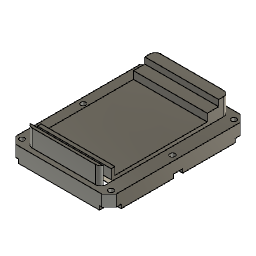
1006315G-Modified (Autodesk Fusion 360 design; units mm, degrees)
Autodesk Fusion 360 part; units mm, degrees
sketch "Sketch1" plane through (0, 0, 0) normal (0, 0, 1) x (1, 0, 0)
  line L0 (6.096, 0) -> (78.105, 0)
  line L1 (84.201, 6.096) -> (84.201, 109.9566)
  line L2 (78.105, 116.0526) -> (6.096, 116.0526)
  line L3 (0, 109.9566) -> (0, 6.096)
  line L4 (6.096, 116.0526) -> (0, 109.9566)
  line L5 (84.201, 109.9566) -> (78.105, 116.0526)
  line L6 (6.096, 0) -> (0, 6.096)
  line L7 (78.105, 0) -> (84.201, 6.096)
  line L8 (93.6149, 58.0263) -> (74.7871, 58.0263) construction
  line L9 (74.7871, 58.0263) -> (-7.9105, 58.0263) construction
  line L10 (91.1489, 109.5883) -> (-7.9105, 109.5883) construction
  line L11 (91.1489, 6.4643) -> (-4.9152, 6.4643) construction
  line L12 (42.1005, 123.6479) -> (42.1005, 108.4573) construction
  line L13 (42.1005, 108.4573) -> (42.1005, -5.2893) construction
  line L14 (79.4385, 120.5753) -> (79.4385, -5.6753) construction
  line L15 (4.7625, 120.9613) -> (4.7625, -5.2893) construction
  circle A0 centre (4.7625, 57.836) radius 2.159
  circle A1 centre (79.4385, 109.5883) radius 2.159
  circle A2 centre (4.7625, 109.5883) radius 2.159
  circle A3 centre (4.7625, 6.4643) radius 2.159
  circle A4 centre (79.4385, 6.4643) radius 2.159
  line L16 (15.4178, 111.887) -> (68.7578, 111.887)
  line L17 (73.0758, 107.569) -> (73.0758, 8.509)
  line L18 (68.7578, 4.191) -> (15.4178, 4.191)
  line L19 (11.0998, 8.509) -> (11.0998, 107.569)
  arc A5 (15.4178, 111.887) -> (11.0998, 107.569) centre (15.4178, 107.569) ccw
  arc A6 (73.0758, 107.569) -> (68.7578, 111.887) centre (68.7578, 107.569) ccw
  arc A7 (11.0998, 8.509) -> (15.4178, 4.191) centre (15.4178, 8.509) ccw
  arc A8 (68.7578, 4.191) -> (73.0758, 8.509) centre (68.7578, 8.509) ccw
  line L20 (0, 61.8363) -> (6.35, 61.8363)
  line L21 (8.89, 59.2963) -> (8.89, 56.7563)
  line L22 (6.35, 54.2163) -> (0, 54.2163)
  line L23 (0, 54.2163) -> (0, 61.8363)
  arc A9 (8.89, 59.2963) -> (6.35, 61.8363) centre (6.35, 59.2963) ccw
  arc A10 (6.35, 54.2163) -> (8.89, 56.7563) centre (6.35, 56.7563) ccw
  line L24 (84.201, 54.2163) -> (77.851, 54.2163)
  line L25 (75.311, 56.7563) -> (75.311, 59.2963)
  line L26 (77.851, 61.8363) -> (84.201, 61.8363)
  line L27 (84.201, 61.8363) -> (84.201, 54.2163)
  circle A11 centre (79.4385, 58.0263) radius 2.159
  arc A12 (77.851, 61.8363) -> (75.311, 59.2963) centre (77.851, 59.2963) ccw
  arc A13 (75.311, 56.7563) -> (77.851, 54.2163) centre (77.851, 56.7563) ccw
  line L28 (76.073, 0) -> (84.201, 0)
  line L29 (84.201, 0) -> (84.201, 10.16)
  line L30 (84.201, 10.16) -> (78.613, 10.16)
  line L31 (76.073, 7.62) -> (76.073, 0)
  arc A14 (78.613, 10.16) -> (76.073, 7.62) centre (78.613, 7.62) ccw
  line L32 (8.128, 0) -> (0, 0)
  line L33 (0, 0) -> (0, 10.16)
  line L34 (0, 10.16) -> (5.588, 10.16)
  line L35 (8.128, 7.62) -> (8.128, 0)
  arc A15 (8.128, 7.62) -> (5.588, 10.16) centre (5.588, 7.62) ccw
  line L36 (0, 105.8179) -> (5.588, 105.8179)
  line L37 (8.128, 108.3579) -> (8.128, 115.9779)
  line L38 (8.128, 115.9779) -> (0, 115.9779)
  line L39 (0, 115.9779) -> (0, 105.8179)
  arc A16 (5.588, 105.8179) -> (8.128, 108.3579) centre (5.588, 108.3579) ccw
  line L40 (76.073, 116.0526) -> (84.201, 116.0526)
  line L41 (84.201, 116.0526) -> (84.201, 105.8926)
  line L42 (84.201, 105.8926) -> (78.613, 105.8926)
  line L43 (76.073, 108.4326) -> (76.073, 116.0526)
  arc A17 (76.073, 108.4326) -> (78.613, 105.8926) centre (78.613, 108.4326) ccw
  line L44 (11.0998, 103.124) -> (73.0758, 103.124)
  line L45 (11.0998, 6.604) -> (73.0758, 6.604)
  line L46 (11.0998, 12.954) -> (73.0758, 12.954)
  point P0 (84.201, 0)
  point P1 (84.201, 116.0526)
  point P2 (0, 116.0526)
  point P3 (11.0998, 111.887)
  point P4 (73.0758, 111.887)
  point P5 (8.89, 61.8363)
  point P6 (75.311, 61.8363)
  point P7 (76.073, 10.16)
  point P8 (8.128, 10.16)
  point P9 (8.128, 105.8179)
  point P10 (76.073, 105.8926)
  dimension "d1" = 84.201
  dimension "d2" = 116.0526
  dimension "d3" = 6.096
  dimension "d4" = 6.096
  dimension "d5" = 6.096
  dimension "d6" = 6.096
  dimension "d7" = 6.096
  dimension "d8" = 6.096
  dimension "d9" = 6.096
  dimension "d10" = 6.096
  dimension "d11" = 51.562
  dimension "d12" = 51.562
  dimension "d13" = 37.338
  dimension "d14" = 37.338
  dimension "d16" = 4.318
  dimension "d17" = 4.318
  dimension "d18" = 4.318
  dimension "d19" = 4.318
  dimension "d20" = 4.318
  dimension "d21" = 61.976
  dimension "d22" = 11.1252
  dimension "d23" = 107.696
  dimension "d24" = 4.1656
  dimension "d25" = 4.318
  dimension "d26" = 4.318
  dimension "d27" = 4.318
  dimension "d28" = 4.318
  dimension "d33" = 7.62
  dimension "d34" = 8.89
  dimension "d35" = 3.81
  dimension "d36" = 2.54
  dimension "d37" = 2.54
  dimension "d38" = 7.62
  dimension "d39" = 8.89
  dimension "d40" = 3.81
  dimension "d41" = 4.318
  dimension "d42" = 2.54
  dimension "d43" = 2.54
  dimension "d44" = 10.16
  dimension "d45" = 8.128
  dimension "d46" = 2.54
  dimension "d52" = 10.16
  dimension "d53" = 8.128
  dimension "d54" = 2.54
  dimension "d55" = 10.16
  dimension "d56" = 8.128
  dimension "d57" = 2.54
  dimension "d58" = 10.16
  dimension "d59" = 8.128
  dimension "d60" = 2.54
  dimension "d75" = 96.52
  dimension "d77" = 6.35
  dimension "d84" = 8.763
  constraint horizontal L0
  constraint vertical L1
  constraint horizontal L2
  constraint vertical L3
  constraint coincident L32.end L33.start
  constraint coincident P2 L2
  constraint coincident P2 L3
  constraint coincident P1 L1
  constraint coincident P1 L2
  constraint coincident L32.end L0
  constraint coincident L32.end L3
  constraint coincident P0 L0
  constraint coincident P0 L1
  constraint horizontal L8
  constraint midpoint L1 L8
  constraint perpendicular L1 L9
  constraint perpendicular L3 L10
  constraint perpendicular L3 L11
  constraint vertical L12
  constraint midpoint L2 L12
  constraint perpendicular L0 L13
  constraint perpendicular L2 L14
  constraint perpendicular L0 L15
  constraint midpoint L15 A0.centre
  constraint coincident L10 A1.centre
  constraint coincident L14 A1.centre
  constraint coincident L10 A2.centre
  constraint coincident L15 A2.centre
  constraint coincident L11 A3.centre
  constraint coincident L15 A3.centre
  constraint coincident L11 A4.centre
  constraint coincident L14 A4.centre
  constraint horizontal L16
  constraint vertical L17
  constraint horizontal L18
  constraint vertical L19
  constraint coincident P3 L16
  constraint coincident P3 L19
  constraint tangent L16 A5
  constraint tangent L19 A5
  constraint coincident P4 L16
  constraint coincident P4 L17
  constraint tangent L16 A6
  constraint tangent L17 A6
  constraint tangent L18 A7
  constraint tangent L19 A7
  constraint tangent L17 A8
  constraint tangent L18 A8
  constraint horizontal L20
  constraint vertical L21
  constraint horizontal L22
  constraint vertical L23
  constraint coincident L3 L20.start
  constraint coincident P5 L20
  constraint coincident P5 L21
  constraint tangent L20 A9
  constraint tangent L21 A9
  constraint tangent L21 A10
  constraint tangent L22 A10
  constraint horizontal L24
  constraint vertical L25
  constraint horizontal L26
  constraint vertical L27
  constraint coincident L1 L24.start
  constraint coincident L14 A11.centre
  constraint coincident L8 A11.centre
  constraint coincident P6 L25
  constraint coincident P6 L26
  constraint tangent L25 A12
  constraint tangent L26 A12
  constraint tangent L24 A13
  constraint tangent L25 A13
  constraint horizontal L28
  constraint vertical L29
  constraint horizontal L30
  constraint vertical L31
  constraint coincident L0 L28.start
  constraint coincident P7 L30
  constraint coincident P7 L31
  constraint tangent L30 A14
  constraint tangent L31 A14
  constraint horizontal L32
  constraint vertical L33
  constraint horizontal L34
  constraint vertical L35
  constraint coincident L0 L32.start
  constraint coincident P8 L34
  constraint coincident P8 L35
  constraint tangent L34 A15
  constraint tangent L35 A15
  constraint horizontal L36
  constraint vertical L37
  constraint horizontal L38
  constraint vertical L39
  constraint coincident L3 L36.start
  constraint coincident P9 L36
  constraint coincident P9 L37
  constraint tangent L36 A16
  constraint tangent L37 A16
  constraint horizontal L40
  constraint vertical L41
  constraint horizontal L42
  constraint vertical L43
  constraint coincident L2 L40.start
  constraint coincident P10 L42
  constraint coincident P10 L43
  constraint tangent L42 A17
  constraint tangent L43 A17
  constraint coincident L19 L44.start
  constraint coincident L17 L44.end
  constraint perpendicular L17 L44
  constraint coincident L19 L45.start
  constraint coincident L17 L45.end
  constraint perpendicular L17 L45
  constraint coincident L19 L46.start
  constraint coincident L17 L46.end
  constraint perpendicular L17 L46
  measures "d1" distance of L32.end P0
  measures "d2" distance of L32.end P2
  measures "d3" distance of P2 L2.end
  measures "d4" distance of P2 L3.start
  measures "d5" distance of P1 L1.end
  measures "d6" distance of P1 L2.start
  measures "d7" distance of L32.end L0.start
  measures "d8" distance of L32.end L3.end
  measures "d9" distance of P0 L0.end
  measures "d10" distance of P0 L1.start
  measures "d11" distance of L8 L10
  measures "d12" distance of L8 L11
  measures "d13" distance of L13 L14
  measures "d14" distance of L13 L15
  measures "d16" diameter of A0
  measures "d17" diameter of A1
  measures "d18" diameter of A2
  measures "d19" diameter of A3
  measures "d20" diameter of A4
  measures "d21" distance of P3 P4
  measures "d22" distance of L1 L17
  measures "d23" distance of L16 L18
  measures "d24" distance of L2 L16
  measures "d25" radius of A5
  measures "d26" radius of A6
  measures "d27" radius of A7
  measures "d28" radius of A8
  measures "d33" distance of L20.start L22.end
  measures "d34" distance of L20.start P5
  measures "d35" distance of L9 L20
  measures "d36" radius of A9
  measures "d37" radius of A10
  measures "d38" distance of L24.start L26.end
  measures "d39" distance of P6 L26.end
  measures "d40" distance of L8 L24
  measures "d41" diameter of A11
  measures "d42" radius of A12
  measures "d43" radius of A13
  measures "d44" distance of L28.start P7
  measures "d45" distance of L29.end P7
  measures "d46" radius of A14
  measures "d52" distance of L32.start P8
  measures "d53" distance of L33.end P8
  measures "d54" radius of A15
  measures "d55" distance of L36.start L38.end
  measures "d56" distance of L36.start P9
  measures "d57" radius of A16
  measures "d58" distance of L40.start P10
  measures "d59" distance of L41.end P10
  measures "d60" radius of A17
  measures "d75" distance of L44 L45
  measures "d77" distance of L45 L46
  measures "d84" distance of L16 L44
extrude "Extrude1" add sketch "Sketch1" along normal blind 12.7 contours L0 L3 L6 L32 L33 L34 L35 A15 | L0 L1 L2 L3 L4 L20 L21 L22 A9 A10 L24 L25 L26 A12 A13 L30 L31 A14 L34 L35 A15 L36 L37 L38 A16 L42 L43 A17 | L0 L1 L7 L28 L29 L30 L31 A14 | L3 L20 L21 L22 L23 A9 A10 | L3 L4 L36 L37 L38 L39 A16 | L1 L24 L25 L26 L27 A12 A13 | L1 L2 L5 L40 L41 L42 L43 A17 | A11
extrude "Extrude2" add sketch "Sketch1" along normal blind 22.098 contours L16 L17 L19 A5 A6 L44 | L17 L19 L44 L46 | L17 L19 A7 A8 L45 L46 | L18 A7 A8 L45
extrude "Extrude3" cut sketch "Sketch1" along normal through all contours A11
extrude "Extrude4" cut sketch "Sketch1" along normal blind 3.175 contours L1 L24 L25 L26 L27 A12 A13
extrude "Extrude5" cut sketch "Sketch1" along normal blind 3.175 contours L0 L1 L7 L28 L29 L30 L31 A14
extrude "Extrude6" cut sketch "Sketch1" along normal blind 3.175 contours L1 L2 L5 L40 L41 L42 L43 A17
extrude "Extrude7" cut sketch "Sketch1" along normal blind 3.175 contours L3 L4 L36 L37 L38 L39 A16
extrude "Extrude8" cut sketch "Sketch1" along normal blind 3.175 contours L0 L3 L6 L32 L33 L34 L35 A15
extrude "Extrude9" cut sketch "Sketch1" along normal blind 3.175 contours L3 L20 L21 L22 L23 A9 A10
sketch "Sketch2" plane through (0, 0, 0) normal (1, 0, 0) x (0, 1, 0)
  line L0 (58.0263, -11.1893) -> (58.0263, 11.1893) construction
  line L1 (6.096, 0) -> (109.9566, 0)
  line L2 (16.1163, 23.368) -> (93.5863, 23.368)
  line L3 (93.5863, 23.368) -> (93.5863, 15.748)
  line L4 (93.5863, 15.748) -> (16.1163, 15.748)
  line L5 (16.1163, 15.748) -> (16.1163, 23.368)
  line L6 (58.0263, 11.1893) -> (58.0263, 27.3313) construction
  line L7 (12.736, 14.3641) -> (23.3597, 0)
  line L8 (12.736, 0) -> (12.736, 14.3641)
  dimension "d70" = 77.47
  dimension "d72" = 7.62
  dimension "d73" = 15.748
  dimension "d85" = 41.91
  constraint vertical L0
  constraint midpoint L0 L1
  constraint horizontal L2
  constraint vertical L3
  constraint horizontal L4
  constraint vertical L5
  constraint perpendicular L4 L6
  constraint coincident L1 L7.end
  constraint coincident L1 L8.start
  measures "d70" distance of L3 L5
  measures "d72" distance of L2.end L3.end
  measures "d73" distance of L1 L4
  measures "d85" distance of L5 L6
extrude "Extrude11" add sketch "Sketch1" along normal blind 27.3304 contours L16 L17 L19 A5 A6 L44
extrude "Extrude12" add sketch "Sketch1" along normal blind 27.3304 contours L18 A7 A8 L45
extrude "Extrude13" cut sketch "Sketch1" along normal through all contours L17 L19 A7 A8 L45 L46
extrude "Extrude14" cut sketch "Sketch2" along normal through all contours L2 L3 L4 L5
extrude "Extrude15" cut sketch "Sketch2" along normal blind 61.976 from surface at 11.1252 contours L1 L7 L8
equation "d4 = d3"
equation "d6 = d5"
equation "d8 = d7"
equation "d10 = d9"
